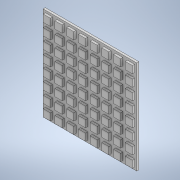
# Autodesk Inventor part: LedMatrix
Saved by Autodesk Inventor 2020.1 (Build 241239000, 239)
## iProperties
Created: 2019-09-02
Part Number: LedMatrix
Material: Generic
Document SubType Name: Modeling
Designer: matteo.spadetto-1
Density: 1 g/cm^3
Appearance: Default
Author: matteo.spadetto-1
Autodesk Inventor part; units mm, degrees
ref_plane "YZ Plane" through (0, 0, 0) normal (1, 0, 0) x (0, 1, 0)
ref_plane "XZ Plane" through (0, 0, 0) normal (0, 1, 0) x (-1, 0, 0)
ref_plane "XY Plane" through (0, 0, 0) normal (0, 0, 1) x (1, 0, 0)
sketch "Sketch2" plane through (0, 0, 0) normal (0, 0, 1) x (1, 0, 0)
  line L0 (0, 0) -> (65, 0)
  line L1 (65, 0) -> (65, 65)
  line L2 (65, 65) -> (0, 65)
  line L3 (0, 65) -> (0, 0)
  dimension "d0" = 65
  dimension "d1" = 65
  constraints: 8 end point, 2 parallel, 1 horizontal, 1 perpendicular
  measures "d0" distance of L2.end L1.end
  measures "d1" distance of L1.end L0.end
extrude "Extrusion1" add sketch "Sketch2" along normal blind 1.5
sketch "Sketch3" plane through (0, 0, 1.5) normal (0, 0, 1) x (1, 0, 0)
  line L0 (65, 65) -> (0, 65) projected
  line L1 (65, 0) -> (65, 65) projected
  line L2 (0, 65) -> (6.562, 65)
  line L3 (65, 65) -> (65, 0)
  line L4 (65, 0) -> (63.43, 0)
  line L5 (0, 0) -> (0, 22.818)
  line L6 (1.562, 63.438) -> (1.562, 58.438)
  line L7 (1.562, 55.314) -> (1.562, 50.314)
  line L8 (1.562, 39.066) -> (1.562, 34.066)
  line L9 (1.562, 30.942) -> (1.562, 25.942)
  line L10 (1.562, 14.694) -> (1.562, 9.694)
  line L11 (1.562, 6.57) -> (1.562, 1.57)
  line L12 (1.562, 0) -> (0, 0)
  line L13 (0, 63.438) -> (0, 65)
  line L14 (0, 58.438) -> (0, 63.438)
  line L15 (0, 55.314) -> (0, 58.438)
  line L16 (0, 42.19) -> (0, 55.314)
  line L17 (0, 34.066) -> (0, 42.19)
  line L18 (0, 25.942) -> (0, 34.066)
  line L19 (0, 22.818) -> (0, 25.942)
  line L20 (6.562, 65) -> (9.686, 65)
  line L21 (6.562, 63.438) -> (6.562, 58.438)
  line L22 (6.562, 55.314) -> (6.562, 50.314)
  line L23 (6.562, 30.942) -> (6.562, 25.942)
  line L24 (6.562, 22.818) -> (6.562, 17.818)
  line L25 (6.562, 14.694) -> (6.562, 9.694)
  line L26 (6.562, 6.57) -> (6.562, 1.57)
  line L27 (9.686, 65) -> (14.686, 65)
  line L28 (9.686, 47.19) -> (9.686, 42.19)
  line L29 (9.686, 30.942) -> (9.686, 25.942)
  line L30 (9.686, 22.818) -> (14.686, 22.818)
  line L31 (9.686, 17.818) -> (14.686, 17.818)
  line L32 (9.686, 14.694) -> (14.686, 14.694)
  line L33 (9.686, 1.57) -> (14.686, 1.57)
  line L34 (14.686, 65) -> (42.182, 65)
  line L35 (14.686, 55.314) -> (14.686, 50.314)
  line L36 (14.686, 47.19) -> (14.686, 42.19)
  line L37 (14.686, 39.066) -> (14.686, 34.066)
  line L38 (14.686, 30.942) -> (14.686, 25.942)
  line L39 (17.81, 55.314) -> (17.81, 50.314)
  line L40 (17.81, 39.066) -> (22.81, 39.066)
  line L41 (17.81, 30.942) -> (17.81, 25.942)
  line L42 (17.81, 14.694) -> (22.81, 14.694)
  line L43 (17.81, 6.57) -> (17.81, 1.57)
  line L44 (22.81, 63.438) -> (22.81, 58.438)
  line L45 (22.81, 55.314) -> (22.81, 50.314)
  line L46 (22.81, 47.19) -> (22.81, 42.19)
  line L47 (22.81, 22.818) -> (22.81, 17.818)
  line L48 (22.81, 6.57) -> (22.81, 1.57)
  line L49 (25.934, 55.314) -> (25.934, 50.314)
  line L50 (25.934, 39.066) -> (30.934, 39.066)
  line L51 (25.934, 30.942) -> (25.934, 25.942)
  line L52 (25.934, 22.818) -> (25.934, 17.818)
  line L53 (25.934, 14.694) -> (25.934, 9.694)
  line L54 (25.934, 6.57) -> (25.934, 1.57)
  line L55 (25.934, 0) -> (1.562, 0)
  line L56 (30.934, 22.818) -> (30.934, 17.818)
  line L57 (30.934, 63.438) -> (30.934, 58.438)
  line L58 (34.058, 55.314) -> (34.058, 50.314)
  line L59 (34.058, 47.19) -> (34.058, 42.19)
  line L60 (34.058, 30.942) -> (34.058, 25.942)
  line L61 (34.058, 14.694) -> (39.058, 14.694)
  line L62 (34.058, 1.57) -> (39.058, 1.57)
  line L63 (39.058, 55.314) -> (39.058, 50.314)
  line L64 (39.058, 30.942) -> (39.058, 25.942)
  line L65 (39.058, 22.818) -> (39.058, 17.818)
  line L66 (42.182, 65) -> (47.182, 65)
  line L67 (42.182, 58.438) -> (47.182, 58.438)
  line L68 (42.182, 55.314) -> (42.182, 50.314)
  line L69 (42.182, 47.19) -> (42.182, 42.19)
  line L70 (42.182, 39.066) -> (42.182, 34.066)
  line L71 (42.182, 30.942) -> (42.182, 25.942)
  line L72 (47.182, 65) -> (58.43, 65)
  line L73 (47.182, 47.19) -> (47.182, 42.19)
  line L74 (47.182, 39.066) -> (47.182, 34.066)
  line L75 (47.182, 14.694) -> (47.182, 9.694)
  line L76 (47.182, 6.57) -> (47.182, 1.57)
  line L77 (47.182, 0) -> (25.934, 0)
  line L78 (50.306, 58.438) -> (55.306, 58.438)
  line L79 (50.306, 55.314) -> (55.306, 55.314)
  line L80 (50.306, 47.19) -> (50.306, 42.19)
  line L81 (50.306, 34.066) -> (55.306, 34.066)
  line L82 (50.306, 17.818) -> (55.306, 17.818)
  line L83 (50.306, 14.694) -> (50.306, 9.694)
  line L84 (50.306, 0) -> (47.182, 0)
  line L85 (55.306, 47.19) -> (55.306, 42.19)
  line L86 (55.306, 30.942) -> (55.306, 25.942)
  line L87 (58.43, 63.438) -> (58.43, 58.438)
  line L88 (58.43, 63.438) -> (63.43, 63.438)
  line L89 (58.43, 55.314) -> (58.43, 50.314)
  line L90 (58.43, 47.19) -> (58.43, 42.19)
  line L91 (58.43, 39.066) -> (58.43, 34.066)
  line L92 (58.43, 22.818) -> (58.43, 17.818)
  line L93 (58.43, 9.694) -> (63.43, 9.694)
  line L94 (58.43, 1.57) -> (63.43, 1.57)
  line L95 (63.43, 47.19) -> (63.43, 42.19)
  line L96 (63.43, 0) -> (50.306, 0)
  line L97 (58.43, 65) -> (65, 65)
  line L98 (1.562, 63.438) -> (6.562, 63.438)
  line L99 (9.686, 63.438) -> (14.686, 63.438)
  line L100 (17.81, 63.438) -> (22.81, 63.438)
  line L101 (25.934, 63.438) -> (30.934, 63.438)
  line L102 (34.058, 63.438) -> (39.058, 63.438)
  line L103 (42.182, 63.438) -> (47.182, 63.438)
  line L104 (50.306, 63.438) -> (55.306, 63.438)
  line L105 (39.058, 58.438) -> (34.058, 58.438)
  line L106 (30.934, 58.438) -> (25.934, 58.438)
  line L107 (22.81, 58.438) -> (17.81, 58.438)
  line L108 (14.686, 58.438) -> (9.686, 58.438)
  line L109 (6.562, 58.438) -> (1.562, 58.438)
  line L110 (58.43, 58.438) -> (63.43, 58.438)
  line L111 (58.43, 50.314) -> (63.43, 50.314)
  line L112 (55.306, 50.314) -> (50.306, 50.314)
  line L113 (47.182, 50.314) -> (42.182, 50.314)
  line L114 (39.058, 50.314) -> (34.058, 50.314)
  line L115 (30.934, 50.314) -> (25.934, 50.314)
  line L116 (22.81, 50.314) -> (17.81, 50.314)
  line L117 (14.686, 50.314) -> (9.686, 50.314)
  line L118 (6.562, 50.314) -> (1.562, 50.314)
  line L119 (47.182, 55.314) -> (42.182, 55.314)
  line L120 (39.058, 55.314) -> (34.058, 55.314)
  line L121 (30.934, 55.314) -> (25.934, 55.314)
  line L122 (22.81, 55.314) -> (17.81, 55.314)
  line L123 (14.686, 55.314) -> (9.686, 55.314)
  line L124 (6.562, 55.314) -> (1.562, 55.314)
  line L125 (9.686, 47.19) -> (14.686, 47.19)
  line L126 (17.81, 47.19) -> (22.81, 47.19)
  line L127 (25.934, 47.19) -> (30.934, 47.19)
  line L128 (34.058, 47.19) -> (39.058, 47.19)
  line L129 (42.182, 47.19) -> (47.182, 47.19)
  line L130 (50.306, 47.19) -> (55.306, 47.19)
  line L131 (58.43, 47.19) -> (63.43, 47.19)
  line L132 (1.562, 47.19) -> (6.562, 47.19)
  line L133 (14.686, 42.19) -> (9.686, 42.19)
  line L134 (25.934, 42.19) -> (30.934, 42.19)
  line L135 (17.81, 42.19) -> (22.81, 42.19)
  line L136 (34.058, 42.19) -> (39.058, 42.19)
  line L137 (42.182, 42.19) -> (47.182, 42.19)
  line L138 (50.306, 42.19) -> (55.306, 42.19)
  line L139 (58.43, 42.19) -> (63.43, 42.19)
  line L140 (6.562, 42.19) -> (1.562, 42.19)
  line L141 (14.686, 39.066) -> (9.686, 39.066)
  line L142 (6.562, 39.066) -> (1.562, 39.066)
  line L143 (34.058, 39.066) -> (39.058, 39.066)
  line L144 (42.182, 39.066) -> (47.182, 39.066)
  line L145 (50.306, 39.066) -> (55.306, 39.066)
  line L146 (58.43, 39.066) -> (63.43, 39.066)
  line L147 (58.43, 34.066) -> (63.43, 34.066)
  line L148 (47.182, 34.066) -> (42.182, 34.066)
  line L149 (39.058, 34.066) -> (34.058, 34.066)
  line L150 (30.934, 34.066) -> (25.934, 34.066)
  line L151 (22.81, 34.066) -> (17.81, 34.066)
  line L152 (14.686, 34.066) -> (9.686, 34.066)
  line L153 (6.562, 34.066) -> (1.562, 34.066)
  line L154 (1.562, 30.942) -> (6.562, 30.942)
  line L155 (9.686, 30.942) -> (14.686, 30.942)
  line L156 (17.81, 30.942) -> (22.81, 30.942)
  line L157 (25.934, 30.942) -> (30.934, 30.942)
  line L158 (34.058, 30.942) -> (39.058, 30.942)
  line L159 (42.182, 30.942) -> (47.182, 30.942)
  line L160 (50.306, 30.942) -> (55.306, 30.942)
  line L161 (58.43, 30.942) -> (63.43, 30.942)
  line L162 (22.81, 25.942) -> (17.81, 25.942)
  line L163 (14.686, 25.942) -> (9.686, 25.942)
  line L164 (6.562, 25.942) -> (1.562, 25.942)
  line L165 (25.934, 25.942) -> (30.934, 25.942)
  line L166 (34.058, 25.942) -> (39.058, 25.942)
  line L167 (42.182, 25.942) -> (47.182, 25.942)
  line L168 (50.306, 25.942) -> (55.306, 25.942)
  line L169 (58.43, 25.942) -> (63.43, 25.942)
  line L170 (6.562, 22.818) -> (1.562, 22.818)
  line L171 (17.81, 22.818) -> (22.81, 22.818)
  line L172 (25.934, 22.818) -> (30.934, 22.818)
  line L173 (34.058, 22.818) -> (39.058, 22.818)
  line L174 (42.182, 22.818) -> (47.182, 22.818)
  line L175 (50.306, 22.818) -> (55.306, 22.818)
  line L176 (58.43, 22.818) -> (63.43, 22.818)
  line L177 (17.81, 17.818) -> (22.81, 17.818)
  line L178 (25.934, 17.818) -> (30.934, 17.818)
  line L179 (34.058, 17.818) -> (39.058, 17.818)
  line L180 (42.182, 17.818) -> (47.182, 17.818)
  line L181 (58.43, 17.818) -> (63.43, 17.818)
  line L182 (6.562, 17.818) -> (1.562, 17.818)
  line L183 (6.562, 14.694) -> (1.562, 14.694)
  line L184 (25.934, 14.694) -> (30.934, 14.694)
  line L185 (42.182, 14.694) -> (47.182, 14.694)
  line L186 (50.306, 14.694) -> (55.306, 14.694)
  line L187 (58.43, 14.694) -> (63.43, 14.694)
  line L188 (55.306, 9.694) -> (50.306, 9.694)
  line L189 (47.182, 9.694) -> (42.182, 9.694)
  line L190 (39.058, 9.694) -> (34.058, 9.694)
  line L191 (30.934, 9.694) -> (25.934, 9.694)
  line L192 (22.81, 9.694) -> (17.81, 9.694)
  line L193 (14.686, 9.694) -> (9.686, 9.694)
  line L194 (6.562, 9.694) -> (1.562, 9.694)
  line L195 (6.562, 1.57) -> (1.562, 1.57)
  line L196 (17.81, 1.57) -> (22.81, 1.57)
  line L197 (25.934, 1.57) -> (30.934, 1.57)
  line L198 (42.182, 1.57) -> (47.182, 1.57)
  line L199 (50.306, 1.57) -> (55.306, 1.57)
  line L200 (50.306, 6.57) -> (55.306, 6.57)
  line L201 (58.43, 6.57) -> (63.43, 6.57)
  line L202 (39.058, 6.57) -> (34.058, 6.57)
  line L203 (30.934, 6.57) -> (25.934, 6.57)
  line L204 (22.81, 6.57) -> (17.81, 6.57)
  line L205 (14.686, 6.57) -> (9.686, 6.57)
  line L206 (6.562, 6.57) -> (1.562, 6.57)
  line L207 (42.182, 6.57) -> (47.182, 6.57)
  line L208 (9.686, 6.57) -> (9.686, 1.57)
  line L209 (14.686, 6.57) -> (14.686, 1.57)
  line L210 (30.934, 6.57) -> (30.934, 1.57)
  line L211 (34.058, 6.57) -> (34.058, 1.57)
  line L212 (39.058, 6.57) -> (39.058, 1.57)
  line L213 (42.182, 1.57) -> (42.182, 6.57)
  line L214 (50.306, 6.57) -> (50.306, 1.57)
  line L215 (55.306, 6.57) -> (55.306, 1.57)
  line L216 (58.43, 6.57) -> (58.43, 1.57)
  line L217 (63.43, 6.57) -> (63.43, 1.57)
  line L218 (63.43, 14.694) -> (63.43, 9.694)
  line L219 (58.43, 14.694) -> (58.43, 9.694)
  line L220 (30.934, 14.694) -> (30.934, 9.694)
  line L221 (34.058, 14.694) -> (34.058, 9.694)
  line L222 (42.182, 14.694) -> (42.182, 9.694)
  line L223 (55.306, 14.694) -> (55.306, 9.694)
  line L224 (9.686, 9.694) -> (9.686, 14.694)
  line L225 (14.686, 14.694) -> (14.686, 9.694)
  line L226 (17.81, 14.694) -> (17.81, 9.694)
  line L227 (22.81, 14.694) -> (22.81, 9.694)
  line L228 (39.058, 14.694) -> (39.058, 9.694)
  line L229 (9.686, 22.818) -> (9.686, 17.818)
  line L230 (14.686, 22.818) -> (14.686, 17.818)
  line L231 (17.81, 22.818) -> (17.81, 17.818)
  line L232 (34.058, 22.818) -> (34.058, 17.818)
  line L233 (42.182, 22.818) -> (42.182, 17.818)
  line L234 (50.306, 22.818) -> (50.306, 17.818)
  line L235 (55.306, 17.818) -> (55.306, 22.818)
  line L236 (63.43, 22.818) -> (63.43, 17.818)
  line L237 (1.562, 22.818) -> (1.562, 17.818)
  line L238 (22.81, 30.942) -> (22.81, 25.942)
  line L239 (30.934, 30.942) -> (30.934, 25.942)
  line L240 (47.182, 30.942) -> (47.182, 25.942)
  line L241 (58.43, 30.942) -> (58.43, 25.942)
  line L242 (47.182, 22.818) -> (47.182, 17.818)
  line L243 (6.562, 39.066) -> (6.562, 34.066)
  line L244 (9.686, 39.066) -> (9.686, 34.066)
  line L245 (17.81, 39.066) -> (17.81, 34.066)
  line L246 (22.81, 39.066) -> (22.81, 34.066)
  line L247 (1.562, 47.19) -> (1.562, 42.19)
  line L248 (17.81, 42.19) -> (17.81, 47.19)
  line L249 (25.934, 34.066) -> (25.934, 39.066)
  line L250 (30.934, 39.066) -> (30.934, 34.066)
  line L251 (34.058, 39.066) -> (34.058, 34.066)
  line L252 (39.058, 39.066) -> (39.058, 34.066)
  line L253 (50.306, 39.066) -> (50.306, 34.066)
  line L254 (50.306, 30.942) -> (50.306, 25.942)
  line L255 (63.43, 25.942) -> (63.43, 30.942)
  line L256 (55.306, 39.066) -> (55.306, 34.066)
  line L257 (63.43, 39.066) -> (63.43, 34.066)
  line L258 (25.934, 47.19) -> (25.934, 42.19)
  line L259 (39.058, 47.19) -> (39.058, 42.19)
  line L260 (6.562, 42.19) -> (6.562, 47.19)
  line L261 (30.934, 47.19) -> (30.934, 42.19)
  line L262 (30.934, 50.314) -> (30.934, 55.314)
  line L263 (9.686, 55.314) -> (9.686, 50.314)
  line L264 (9.686, 58.438) -> (9.686, 63.438)
  line L265 (14.686, 63.438) -> (14.686, 58.438)
  line L266 (17.81, 58.438) -> (17.81, 63.438)
  line L267 (25.934, 63.438) -> (25.934, 58.438)
  line L268 (34.058, 58.438) -> (34.058, 63.438)
  line L269 (39.058, 63.438) -> (39.058, 58.438)
  line L270 (42.182, 63.438) -> (42.182, 58.438)
  line L271 (47.182, 63.438) -> (47.182, 58.438)
  line L272 (47.182, 55.314) -> (47.182, 50.314)
  line L273 (50.306, 55.314) -> (50.306, 50.314)
  line L274 (55.306, 55.314) -> (55.306, 50.314)
  line L275 (50.306, 58.438) -> (50.306, 63.438)
  line L276 (55.306, 63.438) -> (55.306, 58.438)
  line L277 (63.43, 63.438) -> (63.43, 58.438)
  line L278 (58.43, 55.314) -> (63.43, 55.314)
  line L279 (63.43, 55.314) -> (63.43, 50.314)
  constraints: 556 end point, 95 parallel, 78 vertical, 55 collinear, 39 point on line, 37 horizontal, 15 perpendicular
extrude "Extrusion2" add sketch "Sketch3" along normal blind 1.5 contours L98 L21 L109 L6 | L124 L22 L118 L7 | L142 L243 L153 L8 | L154 L23 L164 L9 | L183 L25 L194 L10 | L206 L26 L195 L11 | L24 L182 L237 L170 | L125 L36 L133 L28 | L155 L38 L163 L29 | L30 L230 L31 L229 | L32 L225 L193 L224 | L208 L205 L209 L33 | L35 L117 L263 L123 | L37 L152 L244 L141 | L122 L45 L116 L39 | L40 L246 L151 L245 | L156 L238 L162 L41 | L42 L227 L192 L226 | L204 L48 L196 L43 | L44 L107 L266 L100 | L46 L135 L248 L126 | L47 L177 L231 L171 | L121 L262 L115 L49 | L50 L250 L150 L249 | L157 L239 L165 L51 | L172 L56 L178 L52 | L184 L220 L191 L53 | L203 L210 L197 L54 | L57 L106 L267 L101 | L120 L63 L114 L58 | L128 L259 L136 L59 | L158 L64 L166 L60 | L61 L228 L190 L221 | L211 L202 L212 L62 | L65 L179 L232 L173 | L270 L103 L271 L67 | L119 L272 L113 L68 | L129 L73 L137 L69 | L144 L74 L148 L70 | L159 L240 L167 L71 | L75 L189 L222 L185 | L76 L198 L213 L207 | L275 L104 L276 L78 | L79 L274 L112 L273 | L130 L85 L138 L80 | L253 L145 L256 L81 | L234 L175 L235 L82 | L186 L223 L188 L83 | L86 L168 L254 L160 | L88 L277 L110 L87 | L278 L279 L111 L89 | L131 L95 L139 L90 | L146 L257 L147 L91 | L176 L236 L181 L92 | L219 L187 L218 L93 | L216 L201 L217 L94 | L99 L265 L108 L264 | L102 L269 L105 L268 | L127 L261 L134 L258 | L132 L260 L140 L247 | L143 L252 L149 L251 | L161 L255 L169 L241 | L174 L242 L180 L233 | L214 L200 L215 L199
body "Solid1"
